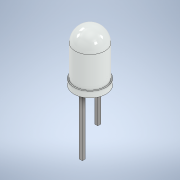
# Autodesk Inventor part: LED
Saved by Autodesk Inventor 2022 (Build 260153000, 153)
## iProperties
Created: 2022-05-23
Part Number: LED
Material: 일반
Document SubType Name: Modeling
Designer: user
Density: 1 g/cm^3
Appearance: 기본값
Author: user
Autodesk Inventor part; units mm, degrees
ref_plane "YZ Plane" through (0, 0, 0) normal (1, 0, 0) x (0, 1, 0)
ref_plane "XZ Plane" through (0, 0, 0) normal (0, 1, 0) x (-1, 0, 0)
ref_plane "XY Plane" through (0, 0, 0) normal (0, 0, 1) x (1, 0, 0)
sketch "스케치1" plane through (0, 0, 0) normal (0, 0, 1) x (1, 0, 0)
  line L0 (0, 0) -> (2.5, 0)
  line L1 (0, 0) -> (0, 8.7)
  line L2 (2.5, 0) -> (2.7, 0)
  line L3 (2.7, 0) -> (2.7, 1)
  line L4 (2.7, 1) -> (2.5, 1)
  line L5 (2.5, 1) -> (2.5, 6.2)
  line L6 (2.5, 8.7) -> (0, 8.7)
  arc A0 (2.5, 6.2) -> (0, 8.7) centre (0, 6.2) ccw
  dimension "d0" = 2.5
  dimension "d1" = 8.7
  dimension "d2" = 0.2
  dimension "d3" = 1
  dimension "d4" = 2.5
  constraints: 14 end point, 4 perpendicular, 2 horizontal, 2 point on circle, 1 centre point, 1 point on line, 1 tangent, 1 vertical
  measures "d0" distance of L0.start L0.end
  measures "d1" distance of L0.start L1.end
  measures "d2" distance of L0.end L2.end
  measures "d3" distance of L2.end L3.end
  measures "d4" distance from line of L6 A0.centre
revolve "회전1" add sketch "스케치1" angle 360 about axis through (0, 0, 0) along (0, 1, 0)
sketch "스케치2" plane through (0, 0, 0) normal (1, 0, 0) x (0, 1, 0)
  line L0 (0, 2.7) -> (0, -2.7) projected
  line L1 (0, -1.56) -> (-6.3813, -1.56)
  line L2 (-6.3813, -1.56) -> (-6.3813, -1.06)
  line L3 (-6.3813, -1.06) -> (0, -1.06)
  line L4 (0, -1.06) -> (0, -1.56)
  line L5 (0, 1.56) -> (-10.1722, 1.56)
  line L6 (-10.1722, 1.56) -> (-10.1722, 1.06)
  line L7 (-10.1722, 1.06) -> (0, 1.06)
  line L8 (0, 1.06) -> (0, 1.56)
  point P0 (0, 0)
  point P1 (0, 1.06)
  dimension "d7" = 1.14
  dimension "d8" = 1.14
  dimension "d9" = 0.5
  dimension "d10" = 0.5
  constraints: 16 end point, 4 parallel, 2 horizontal, 2 perpendicular, 2 point on line
  measures "d7" distance from line of L0.start L5
  measures "d8" distance from line of L1 L0.end
  measures "d9" distance of L1.end L2.end
  measures "d10" distance of L5.end L6.end
extrude "돌출1" add sketch "스케치2" along normal mid plane 0.5
